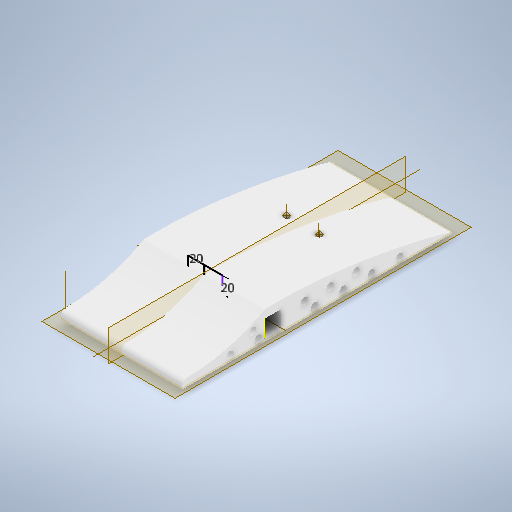
# Autodesk Inventor part: WingBox
Saved by Autodesk Inventor 2026 (Build 300175050, 175E)
## iProperties
Created: 2025-08-01
Part Number: WingBox
Material: Plastic, Opaque White
Document SubType Name: Modeling
Designer: Cupri
Density: 0.952 g/cm^3
Appearance: Smooth - White
Mass: 897.987 g
Surface Area: 1354.71 cm^2
Volume: 943.263 cm^3
Author: Cupri
## iProperties of the stored document WingBox_3DPrint.ipt
Created: 2025-08-03
Part Number: WingBox_3DPrint
Material: Generic
Document SubType Name: Modeling
Designer: Cupri
Density: 1 g/cm^3
Appearance: Default
Author: Cupri
Autodesk Inventor part; units mm, degrees
ref_plane "YZ Plane" through (0, 0, 0) normal (1, 0, 0) x (0, 1, 0)
ref_plane "XY Plane" through (0, 0, 0) normal (0, 0, 1) x (1, 0, 0)
sketch "Sketch1" plane through (0, 0, 0) normal (1, 0, 0) x (0, 1, 0)
  line L0 (-2.1632, -329.9963) -> (-0.9745, -330.0014)
  line L1 (-2.1632, -329.9951) -> (-2.1632, -329.9963)
  line L2 (-2.1632, -329.9951) -> (-2.4422, -329.9951)
  spline S0 degree 3 poles (-0.405, -330.1552) (0.9537, -325.1233) (1.9563, -321.5105) (2.8807, -318.1296) (3.8079, -314.7389) (4.6565, -311.5815) (5.583, -307.9714) (6.5095, -304.3611) (7.5137, -300.2982) (8.6298, -295.6026) (9.7548, -290.8694) (10.9937, -285.4924) (12.2548, -279.8086) (13.5479, -273.9809) (14.8422, -267.9178) (16.0284, -262.0542) (17.2338, -256.0958) (18.3276, -250.3438) (19.3395, -244.7228) (20.6698, -237.333) (21.892, -230.0631) (23.0732, -222.6141) (24.654, -212.6457) (26.1278, -202.3745) (27.3659, -192.1289) (28.2425, -184.8742) (29.0102, -177.6615) (29.6986, -170.63) (30.3698, -163.7739) (30.9693, -157.1031) (31.4539, -150.2338) (31.8154, -145.1091) (32.1063, -139.8058) (32.3036, -134.2671) (32.5007, -128.7338) (32.6046, -122.9656) (32.6262, -117.43) (32.6455, -112.4952) (32.603, -107.8232) (32.5118, -103.6944) (32.4197, -99.5266) (32.278, -95.9127) (32.0844, -92.603) (31.8816, -89.1345) (31.6185, -85.9081) (31.2933, -82.5398) (30.931, -78.7879) (30.4919, -74.8552) (30.0019, -70.9506) (29.515, -67.0719) (28.9863, -63.3007) (28.3579, -59.5488) (27.8334, -56.4177) (27.2229, -53.2286) (26.4972, -49.8793) (25.6301, -45.8774) (24.5968, -41.6418) (23.6015, -37.941) (22.8353, -35.0925) (22.1029, -32.6059) (21.4229, -30.4603) (20.5882, -27.827) (19.838, -25.6271) (18.984, -23.281) (18.321, -21.4595) (17.5736, -19.5423) (16.6309, -17.484) (15.7038, -15.4598) (14.5791, -13.2961) (13.5588, -11.4077) (12.7581, -9.9257) (12.0684, -8.6632) (11.4412, -7.6048) (10.7635, -6.4611) (10.1286, -5.5191) (9.1146, -4.4162) (8.2619, -3.4886) (7.1303, -2.4284) (5.764, -1.4444) (4.4879, -0.5254) (3.0248, 0.2881) (1.5908, 0.5476) (0.3755, 0.7675) (-0.8188, 0.5632) (-1.8076, 0.0108) (-3.0331, -0.6739) (-3.9409, -1.785) (-4.6412, -2.8204) (-5.3573, -3.879) (-5.8545, -4.8644) (-6.2513, -5.8012) (-6.7038, -6.8694) (-7.0446, -7.9661) (-7.4083, -9.3616) (-7.9306, -11.3656) (-8.5009, -13.9974) (-8.9016, -16.5042) (-9.2532, -18.7033) (-9.4614, -20.7666) (-9.6076, -22.6841) (-9.8004, -25.2116) (-9.9342, -27.5205) (-10.0673, -30.276) (-10.1703, -32.4093) (-10.2532, -34.8679) (-10.2982, -37.6909) (-10.3544, -41.2137) (-10.3539, -45.2486) (-10.3194, -49.0894) (-10.289, -52.4587) (-10.2331, -55.6701) (-10.1531, -58.7874) (-10.0605, -62.4007) (-9.9312, -65.9923) (-9.7768, -69.6992) (-9.6107, -73.6891) (-9.4198, -77.7513) (-9.2427, -81.6143) (-9.0879, -84.9923) (-8.9437, -88.2148) (-8.7967, -91.6207) (-8.6574, -94.8459) (-8.5102, -98.3178) (-8.3389, -102.3319) (-8.1674, -106.351) (-7.9717, -110.9139) (-7.7658, -115.7923) (-7.5352, -121.2588) (-7.2978, -127.0252) (-7.0821, -132.579) (-6.8662, -138.1406) (-6.672, -143.4886) (-6.4924, -148.6356) (-6.2558, -155.4121) (-6.0346, -161.9593) (-5.7967, -168.6776) (-5.4813, -177.5831) (-5.1373, -186.7926) (-4.8158, -196.0325) (-4.5204, -204.5215) (-4.2474, -213.0024) (-4.0058, -221.2906) (-3.7869, -228.8022) (-3.5917, -236.1329) (-3.4197, -243.5699) (-3.2893, -249.2072) (-3.1723, -254.9654) (-3.0688, -260.9509) (-2.9665, -266.8676) (-2.8774, -273.0072) (-2.8015, -278.9371) (-2.7285, -284.6426) (-2.6679, -290.0685) (-2.6193, -294.8554) (-2.5708, -299.6265) (-2.5341, -303.7632) (-2.5074, -307.4316) (-2.4807, -311.1183) (-2.464, -314.3315) (-2.4544, -317.7705) (-2.4448, -321.2094) (-2.4422, -324.8742) (-2.4422, -329.9951) knots 0 0 0 0 0.019596 0.019596 0.019596 0.03925 0.03925 0.03925 0.058905 0.058905 0.058905 0.078717 0.078717 0.078717 0.099031 0.099031 0.099031 0.119673 0.119673 0.119673 0.146811 0.146811 0.146811 0.183127 0.183127 0.183127 0.208842 0.208842 0.208842 0.233915 0.233915 0.233915 0.25262 0.25262 0.25262 0.271307 0.271307 0.271307 0.287966 0.287966 0.287966 0.304782 0.304782 0.304782 0.322404 0.322404 0.322404 0.342033 0.342033 0.342033 0.361532 0.361532 0.361532 0.377805 0.377805 0.377805 0.397248 0.397248 0.397248 0.412214 0.412214 0.412214 0.430582 0.430582 0.430582 0.444843 0.444843 0.444843 0.458868 0.458868 0.458868 0.469875 0.469875 0.469875 0.48177 0.48177 0.48177 0.491774 0.491774 0.491774 0.501117 0.501117 0.501117 0.509034 0.509034 0.509034 0.518847 0.518847 0.518847 0.52888 0.52888 0.52888 0.540322 0.540322 0.540322 0.556753 0.556753 0.556753 0.571169 0.571169 0.571169 0.590171 0.590171 0.590171 0.604883 0.604883 0.604883 0.623242 0.623242 0.623242 0.639347 0.639347 0.639347 0.658015 0.658015 0.658015 0.678109 0.678109 0.678109 0.695679 0.695679 0.695679 0.712317 0.712317 0.712317 0.728976 0.728976 0.728976 0.747644 0.747644 0.747644 0.766338 0.766338 0.766338 0.79095 0.79095 0.79095 0.823575 0.823575 0.823575 0.853549 0.853549 0.853549 0.880715 0.880715 0.880715 0.901306 0.901306 0.901306 0.921661 0.921661 0.921661 0.941246 0.941246 0.941246 0.960766 0.960766 0.960766 0.980383 0.980383 0.980383 1 1 1 1
  line L3 (-0.9745, -330.0014) -> (-0.405, -330.1552)
  line L4 (2.197, -97.3811) -> (2.1281, -117.622)
  line L5 (2.1281, -117.622) -> (22.3958, -117.7088)
  line L6 (22.3958, -117.7088) -> (22.4826, -97.4501)
  line L7 (22.4826, -97.4501) -> (2.197, -97.3811)
  line L8 (-2.4422, -329.9951) -> (-2.4422, -0.3997)
  line L9 (-2.4422, -0.3997) -> (-2.4422, 4.6003)
  line L10 (-2.4422, 4.6003) -> (2.4819, 4.6003)
  arc A0 (7.4818, -0.4128) -> (32.3222, -97.4722) centre (207.4812, -0.9354) ccw
  arc A1 (7.4818, -0.4128) -> (2.4819, 4.6003) centre (2.4819, -0.3997) ccw
  line L11 (22.4826, -97.4501) -> (2.2838, -97.4501)
  line L12 (22.3958, -117.7088) -> (2.2838, -117.7088)
  line L13 (12.3398, -117.7088) -> (12.3398, -97.4156) construction
  line L14 (22.4392, -107.5794) -> (2.1626, -107.5015) construction
  point P0 (7.5578, 4.6003)
  dimension "d12" = 5
  dimension "d13" = 10
  dimension "d14" = 200
  dimension "d15" = 5
  constraints: 30 end point, 5 point on circle, 4 midpoint, 3 horizontal, 2 centre point, 2 tangent, 2 vertical, 1 perpendicular, 1 point on line, 4 other
  measures "d12" distance of L8.end L9.end
  measures "d13" distance of L9.end point (7.558, 4.6)
  measures "d14" radius of A0
  measures "d15" radius of A1
extrude "Extrusion1" add sketch "Sketch1" along normal blind 150 contours L2 L8 S0 A0 L3 L0 | L9 L10 A1 A0 S0
sketch "Sketch4" plane through (0, -2.4422, -329.9951) normal (0, -1, 0) x (1, 0, 0)
  line L0 (0, 232.5451) -> (150, 232.5451) construction
  line L1 (0, 232.5451) -> (0, 212.2864) construction
  line L2 (0, 212.2864) -> (150, 212.2864) construction
  line L3 (150, 232.5451) -> (150, 212.2864) construction
  line L4 (105.25, 232.4157) -> (44.75, 232.4157)
  line L5 (44.75, 232.4157) -> (44.75, 161.9157)
  line L6 (44.75, 161.9157) -> (105.25, 161.9157)
  line L7 (105.25, 161.9157) -> (105.25, 232.4157)
  point P0 (0, 329.9951)
  point P1 (75, 100.2234)
  point P2 (150, 222.4157)
  dimension "d37" = 60.5
  dimension "d38" = 70.5
  dimension "d40" = 30.25
  dimension "d41" = 10
  constraints: 8 end point, 2 parallel, 1 horizontal, 1 midpoint, 1 perpendicular
  measures "d37" distance of L6.end L5.end
  measures "d38" distance of L5.end L4.end
  measures "d40" distance from line of point (75, 100.223) L5
  measures "d41" distance from line of point (150, 222.416) L4
extrude "Extrusion4" cut sketch "Sketch4" against normal blind 5
sketch "Sketch5" plane through (0, -2.4422, -329.9951) normal (0, -1, 0) x (1, 0, 0)
  line L0 (64.875, 161.9157) -> (85.125, 161.9157) projected
  line L1 (85.125, 161.9157) -> (85.125, 6.5707) projected
  line L2 (64.875, 6.5707) -> (85.125, 6.5707) projected
  line L3 (64.875, 6.5707) -> (64.875, 161.9157) projected
  line L4 (85.125, 100.2234) -> (64.875, 100.2234) projected
  line L5 (105.25, 212.3713) -> (105.25, 161.9157) projected
  line L6 (105.25, 161.9157) -> (44.75, 161.9157)
  line L7 (44.75, 161.9157) -> (44.75, 100.2234)
  line L8 (44.75, 100.2234) -> (105.25, 100.2234)
  line L9 (105.25, 100.2234) -> (105.25, 161.9157)
  point P0 (0, 329.9951)
  point P1 (64.875, 100.2234)
  point P2 (85.125, 100.2234)
  constraints: 8 end point, 2 parallel, 1 horizontal, 1 perpendicular
extrude "Extrusion5" cut sketch "Sketch5" against normal blind 5 contours L0 L1 L4 L3 | L3 L8 L7 L6 | L6 L9 L8 L1
sketch "Sketch6" plane through (0, 2.5578, -329.9951) normal (0, -1, 0) x (1, 0, 0)
  circle A0 centre (95, 110.7234) radius 2.75
  line L0 (105.25, 100.2234) -> (44.75, 100.2234) projected
  line L1 (75, 100.2234) -> (75, 232.4157) construction
  line L2 (44.75, 232.4157) -> (105.25, 232.4157) projected
  circle A1 centre (55, 110.7234) radius 2.75
  point P0 (0, 329.9951)
  dimension "d46" = 5.5
  dimension "d48" = 20
  dimension "d49" = 10.5
  constraints: 2 centre point, 2 end point, 2 midpoint, 1 symmetric about line, 1 other
  measures "d46" diameter of A0
  measures "d48" distance from line of L1 A0.centre
  measures "d49" distance from line of L0 A0.centre
hole "Hole1" at (55, 23.5974, -219.2718) direction (0, -1, 0) diameter 5.5 end through all start extended yes counterbore diameter 8.5 counterbore depth 15
hole "Hole2" at (95, 23.5974, -219.2718) direction (0, -1, 0) diameter 5.5 end through all start extended yes counterbore diameter 8.5 counterbore depth 15
ref_plane "Work Plane1" through (75, 0, 0) normal (1, 0, 0) x (0, 0, -1)
sketch "Sketch7" plane through (0, 0, 0) normal (-1, 0, 0) x (0, 0, 1)
  line L0 (-117.6238, 2.5578) -> (-117.7088, 22.3958) projected
  line L1 (-97.3811, 2.197) -> (-97.4501, 22.4826) projected
  line L2 (-117.7088, 22.3958) -> (-97.3811, 2.197) construction
  point P0 (0, 0)
  point P1 (-107.5886, 12.3398)
  constraints: 2 end point, 1 point on line
sketch "Sketch8" plane through (150, 2.197, -97.3811) normal (0, -0.0034028, -0.9999942) x (-1, 0, 0)
  line L0 (150, -1.8099) -> (150, 30.1254) projected
  line L1 (150, 30.1254) -> (0, 30.1254) projected
  line L2 (0, -1.8099) -> (0, 30.1254) projected
  line L3 (150, -1.8099) -> (0, -1.8099) projected
  line L4 (64.875, 20.1693) -> (85.125, 0) construction
  point P0 (150, -2.5284)
  point P1 (75, 10.0847)
  constraints: 2 end point, 1 midpoint, 2 other
sketch "Sketch9" plane through (150, 0, 0) normal (1, 0, 0) x (0, 0, -1)
  line L0 (329.9951, -2.4422) -> (335.7928, -2.4422)
  line L1 (335.7928, -2.4422) -> (335.7928, 0.7272)
  line L2 (335.7928, 0.7272) -> (329.9951, 0.7272)
  line L3 (329.9951, 0.7272) -> (329.9951, -2.4422)
  point P0 (0, 0)
  constraints: 8 end point, 2 parallel, 1 horizontal, 1 perpendicular
extrude "Extrusion6" cut sketch "Sketch9" against normal through all
sketch "Sketch10" plane through (150, 0, 0) normal (1, 0, 0) x (0, 0, -1)
  line L0 (-4.6003, -2.4422) -> (329.9951, -2.4422) projected
  circle A0 centre (54.3246, 4.6042) radius 4.5 projected
  circle A1 centre (82.294, 16.3342) radius 4.5 projected
  circle A2 centre (89.3246, 4.5737) radius 4.5 projected
  circle A3 centre (146.294, 16.2785) radius 4.5 projected
  circle A4 centre (159.3246, 4.5127) radius 4.5 projected
  circle A5 centre (178.294, 16.2506) radius 4.5 projected
  circle A6 centre (194.3246, 4.4823) radius 4.5 projected
  circle A7 centre (229.3246, 4.4518) radius 4.5 projected
  circle A8 centre (264.3245, 4.4213) radius 4.5 projected
  circle A9 centre (210.2938, 16.2268) radius 4.5 projected
  circle A10 centre (178.294, 16.2506) radius 4.75
  circle A11 centre (194.3246, 4.4823) radius 4.75
  circle A12 centre (210.2938, 16.2268) radius 4.75
  circle A13 centre (229.3246, 4.4518) radius 4.75
  circle A14 centre (264.3245, 4.4213) radius 4.75
  circle A15 centre (146.294, 16.2785) radius 4.75
  circle A16 centre (159.3246, 4.5127) radius 4.75
  circle A17 centre (89.3246, 4.5737) radius 4.75
  circle A18 centre (82.294, 16.3342) radius 4.75
  circle A19 centre (54.3246, 4.6042) radius 4.75
  point P0 (0, 0)
  dimension "d94" = 0.25
  dimension "d95" = 0.25
  dimension "d96" = 0.25
  dimension "d97" = 0.25
  dimension "d98" = 0.25
  dimension "d99" = 0.25
  dimension "d100" = 0.25
  dimension "d101" = 0.25
  dimension "d102" = 0.25
  dimension "d103" = 0.25
  constraints: 10 centre point
  measures "d94" radial gap between concentric circles of A5 A10
  measures "d95" radial gap between concentric circles of A6 A11
  measures "d96" radial gap between concentric circles of A9 A12
  measures "d97" radial gap between concentric circles of A7 A13
  measures "d98" radial gap between concentric circles of A8 A14
  measures "d99" radial gap between concentric circles of A3 A15
  measures "d100" radial gap between concentric circles of A4 A16
  measures "d101" radial gap between concentric circles of A2 A17
  measures "d102" radial gap between concentric circles of A1 A18
  measures "d103" radial gap between concentric circles of A0 A19
extrude "Extrusion7" cut sketch "Sketch10" against normal blind 5 contours A0 | A1 | A2 | A3 | A4 | A5 | A6 | A7 | A8 | A9 | A10 | A11 | A12 | A13 | A14 | A15 | A16 | A17 | A18 | A19
mirror "Mirror1" about plane through (75, 0, 0) normal (1, 0, 0) of "Extrusion7"
fillet "Fillet1" radius 4.7 10 edges at (145, 4.5737, -84.5746) (145, 4.4823, -189.5746) (145, 4.4213, -259.5745) (145, 4.5127, -154.5746) (145, 16.3342, -77.544) (145, 16.2785, -141.544) (145, 16.2268, -205.5438) (145, 4.4518, -224.5746) (145, 16.2506, -173.544) (145, 4.6042, -49.5746)
sketch "Sketch11" plane through (0, 0, 0) normal (0, 1, 0) x (-1, 0, 0)
  line L0 (-150, -329.9951) -> (0, -329.9951) projected
  line L1 (-150, 4.6003) -> (-150, -329.9951) projected
  line L2 (0, -329.9951) -> (-150, -329.9951)
  line L3 (-150, -329.9951) -> (-150, -328.9951)
  line L4 (-150, -328.9951) -> (0, -328.9951)
  line L5 (0, -328.9951) -> (0, -329.9951)
  point P0 (0, 0)
  dimension "d104" = 1
  constraints: 8 end point, 2 parallel, 1 horizontal, 1 perpendicular, 1 point on line
  measures "d104" distance of L2.end L3.end
extrude "Extrusion8" cut sketch "Sketch11" along normal mid plane 10
fillet "Fillet2" radius 4.7 10 edges at (5, 4.5737, -84.5746) (5, 4.4823, -189.5746) (5, 4.4213, -259.5745) (5, 4.5127, -154.5746) (5, 16.3342, -77.544) (5, 16.2785, -141.544) (5, 16.2268, -205.5438) (5, 4.4518, -224.5746) (5, 16.2506, -173.544) (5, 4.6042, -49.5746)
sketch "Sketch12" plane through (0, 2.5578, -329.9951) normal (0, -1, 0) x (1, 0, 0)
  line L0 (0, 212.3732) -> (44.75, 212.3732) projected
  line L1 (44.75, 212.3732) -> (44.75, 202.3732)
  line L2 (44.75, 100.2234) -> (44.75, 232.4157) projected
  line L3 (44.75, 202.3732) -> (54.75, 202.3732)
  line L4 (54.75, 202.3732) -> (54.75, 212.3732)
  line L5 (54.75, 212.3732) -> (44.75, 212.3732)
  line L6 (44.75, 212.3713) -> (105.25, 212.3713) projected
  line L7 (105.25, 212.3713) -> (95.25, 212.3713)
  line L8 (95.25, 212.3713) -> (95.25, 202.3713)
  line L9 (95.25, 202.3713) -> (105.25, 202.3713)
  line L10 (105.25, 202.3713) -> (105.25, 212.3713)
  point P0 (0, 329.9951)
  point P1 (85.125, 212.3713)
  dimension "d108" = 10
  dimension "d109" = 10
  dimension "d110" = 10
  dimension "d111" = 10
  constraints: 16 end point, 4 perpendicular, 2 parallel, 1 horizontal, 1 point on line
  measures "d108" distance of L0.end L1.end
  measures "d109" distance of L1.end L3.end
  measures "d110" distance of L9.end L8.end
  measures "d111" distance of L8.end L7.end
extrude "Extrusion9" cut sketch "Sketch12" against normal up to surface surface through (0, 22.4826, -97.4501) normal (0, -0.9999908, 0.0042825)
sketch "Sketch13" plane through (150, 22.4826, -97.4501) normal (0, -0.0034028, -0.9999942) x (-1, 0, 0)
  line L0 (150, -20.2857) -> (150, 0) projected
  line L1 (0, -20.2857) -> (0, 0) projected
  line L2 (0, 0) -> (150, 0)
  line L3 (150, 0) -> (150, -20.2857)
  line L4 (150, -20.2857) -> (0, -20.2857)
  line L5 (0, -20.2857) -> (0, 0)
  line L6 (75, 0) -> (52.5304, 0)
  line L7 (52.5304, 0) -> (52.5304, 20)
  line L8 (52.5304, 20) -> (75, 20)
  line L9 (75, 20) -> (75, 0)
  line L10 (75, 0) -> (95, 0)
  line L11 (95, 0) -> (95, 20)
  line L12 (95, 20) -> (75, 20)
  line L13 (75, 20) -> (75, 0)
  point P0 (150, -22.8141)
  dimension "d114" = 20
  dimension "d115" = 20
  constraints: 24 end point, 6 parallel, 3 horizontal, 3 perpendicular, 1 midpoint, 1 point on line
  measures "d114" distance of L6.end L7.end
  measures "d115" distance of L12.end L11.end
body "Solid1"
